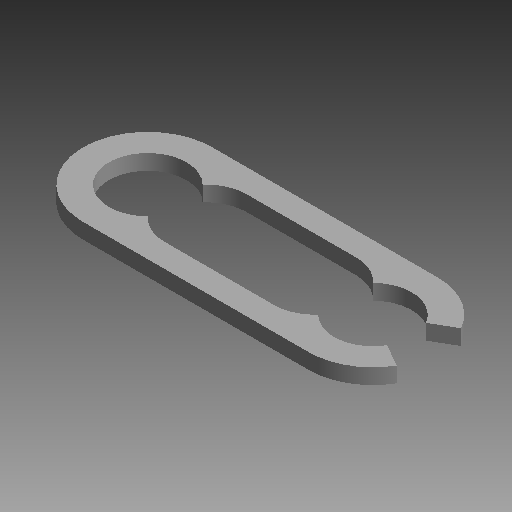
# Autodesk Inventor part: 06B - 1 RP - Clip
Saved by Autodesk Inventor 2019 (Build 230136000, 136)
## iProperties
Category: PARTsolutions
Company: KANA
Part Number: 06B - 1 RP - Clip
Material: 一般
Catalog Web Link: www.cadenas.de
Description: Standard Chain_Clip-
Vendor: KANA
Document SubType Name: Modeling
Designer: partserver
Manufacturer: KANA
Mass: 0.0218026 g
Surface Area: 1.08921 cm^2
Volume: 0.0218026 cm^3
Density: 1 g/cm^3
Appearance: PSOLRGB-192-192-192
PSOL_IDENT_0: {$CADENAS_DATA\23d-libs\kana\roller_chain\standard_chain\standard_chain_clip.prj},187 {VTYP=3D},{NB=
PSOL_IDENT_1: 06B - 1 RP - Clip},{LINA=06B - 1 RP},{NN=Standard Chain_Clip},{DATE=04.07.2018 01:10:23},{GEOMDATE=1
PSOL_IDENT_2: 2.09.2016 07:51:55},{VERSION=},{LINEID=250},{WBVAR=NOL},{WBNUMERIC=NOL}  {NB=06B - 1 RP - Clip},{LIN
PSOL_IDENT_3: A=06B - 1 RP},{KT=DUMMY},{CNO=06B},{PT=RP},{NOL=1},{NOLX=1},{P=9.525},{R=6.350},{W=5.720},{T=1.300},
PSOL_IDENT_4: {H=8.100},{D=3.280},{L=13.6},{C=10.24}
NB: 06B - 1 RP - Clip
NN: Standard Chain_Clip
NBSYN: $CNO. - $NOL. $PT. - Clip
LINA: 06B - 1 RP
CATALOG: KANA
CNO: 06B
PT: RP
NOL: 1
P: 9.525
R: 6.35
W: 5.72
T: 1.3
H: 8.1
D: 3.28
SUPPLIER: KANA
ARTICLENO: 06B - 1 RP - Clip
BOMINFO: 06B - 1 RP
CREATOR: CADENAS GmbH
Title: 06B - 1 RP
Author: Cadenas PARTsolutions
Autodesk Inventor part; units mm, degrees
sketch "Sketch_1" plane through (0, 0, 0) normal (0, 0, 1) x (1, 0, 0)
  arc A0 (-2.3671, -1.3667) -> (0, -2.7333) centre (0, 0) ccw
  line L0 (0, -2.7333) -> (9.525, -2.7333)
  arc A1 (9.525, -2.7333) -> (9.525, 2.7333) centre (9.525, 0) ccw
  line L1 (9.525, 2.7333) -> (0, 2.7333)
  arc A2 (0, 2.7333) -> (-2.3671, 1.3667) centre (0, 0) ccw
  line L2 (-2.3671, 1.3667) -> (-1.4203, 0.82)
  arc A3 (1.1597, 1.1596) -> (-1.4203, 0.82) centre (0, 0) ccw
  arc A4 (2.4548, 1.7384) -> (1.1597, 1.1596) centre (2.4548, 0) ccw
  line L3 (2.4548, 1.7384) -> (7.0702, 1.7384)
  arc A5 (8.3653, 1.1596) -> (7.0702, 1.7384) centre (7.0702, 0) ccw
  arc A6 (8.3653, -1.1596) -> (8.3653, 1.1596) centre (9.525, 0) ccw
  arc A7 (7.0702, -1.7384) -> (8.3653, -1.1596) centre (7.0702, 0) ccw
  line L4 (7.0702, -1.7384) -> (2.4548, -1.7384)
  arc A8 (1.1597, -1.1596) -> (2.4548, -1.7384) centre (2.4548, 0) ccw
  arc A9 (-1.4203, -0.82) -> (1.1597, -1.1596) centre (0, 0) ccw
  line L5 (-1.4203, -0.82) -> (-2.3671, -1.3667)
  constraints: 20 point on circle, 12 end point, 10 centre point
extrude "Extrusion1" add sketch "Sketch_1" along normal blind 0.65
ref_plane "clip_XY" through (0, 0, 0) normal (0, 0, 1) x (1, 0, 0)
ref_plane "clip_YZ" through (0, 0, 0) normal (1, 0, 0) x (0, 1, 0)
ref_plane "clip_ZX" through (0, 0, 0) normal (0, 1, 0) x (0, 0, 1)
body "Solid1"
